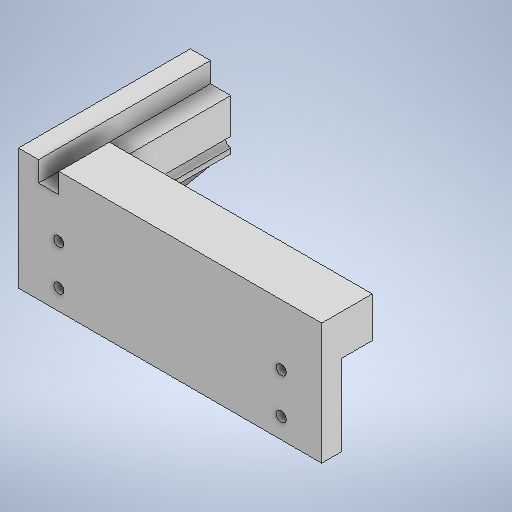
# Autodesk Inventor part: NewModuleConnectorRight
Saved by Autodesk Inventor 2025.3 (Build 293356000, 356)
## iProperties
Created: 2025-05-03
Part Number: NewModuleConnectorRight
Material: 일반
Document SubType Name: Modeling
Designer: SEON
Density: 1 g/cm^3
Appearance: 기본값
Author: SEON
## iProperties of the stored document NewModuleConnectorLeft_3D 인쇄.ipt
Created: 2025-05-03
Part Number: NewModuleConnectorLeft_3D 인쇄
Material: 일반
Document SubType Name: Modeling
Designer: SEON
Density: 1 g/cm^3
Appearance: 기본값
Author: SEON
Autodesk Inventor part; units mm, degrees
ref_plane "YZ Plane" through (0, 0, 0) normal (1, 0, 0) x (0, 1, 0)
ref_plane "XZ Plane" through (0, 0, 0) normal (0, 1, 0) x (-1, 0, 0)
ref_plane "XY Plane" through (0, 0, 0) normal (0, 0, 1) x (1, 0, 0)
sketch "스케치1" plane through (0, 0, 0) normal (0, 0, 1) x (1, 0, 0)
  line L0 (0, 0) -> (150, 0)
  line L1 (150, 0) -> (150, 60)
  line L2 (150, 60) -> (0, 60)
  line L3 (0, 60) -> (0, 0)
  circle A0 centre (20, 30) radius 2.5
  circle A1 centre (20, 10) radius 2.5
  circle A2 centre (130, 30) radius 2.5
  circle A3 centre (130, 10) radius 2.5
  line L4 (10, 60) -> (10, 0)
  line L5 (20, 60) -> (20, 50)
  line L6 (20, 50) -> (10, 50)
  line L7 (20, 50) -> (20, 25)
  line L8 (20, 25) -> (10, 25)
  line L9 (10, 15) -> (0, 15)
  line L10 (20, 40) -> (150, 40)
  point P0 (20, 27.5)
  point P1 (20, 32.5)
  dimension "d0" = 5
  dimension "d1" = 30
  dimension "d2" = 20
  dimension "d3" = 20
  dimension "d4" = 150
  dimension "d5" = 20
  dimension "d6" = 60
  dimension "d7" = 10
  dimension "d8" = 10
  dimension "d9" = 10
  dimension "d10" = 10
  dimension "d11" = 25
  dimension "d16" = 10
  dimension "d19" = 20
  constraints: 22 end point, 9 point on line, 6 perpendicular, 4 centre point, 3 equal radius, 2 horizontal alignment, 2 parallel, 2 vertical alignment, 1 horizontal, 1 vertical
  measures "d0" diameter of A0
  measures "d1" distance from line of L2 A0.centre
  measures "d2" distance of A0.centre A1.centre
  measures "d3" distance from line of A2.centre L1
  measures "d4" distance between parallel lines of L3 L1
  measures "d5" distance from line of L3 A1.centre
  measures "d6" distance of L2.end L0.start
  measures "d7" distance between parallel lines of L3 L4
  measures "d8" distance of L5.end L6.end
  measures "d9" distance of L5.start L5.end
  measures "d10" distance of L7.end L8.end
  measures "d11" distance of L5.end L7.end
  measures "d16" distance between parallel lines of L8 L9
  measures "d19" distance of L1.end L10.end
extrude "돌출1" add sketch "스케치1" along normal blind 10 contours L3 L9 L4 L0 | L4 L8 L7 A0 L10 L1 L0 | L3 L2 L4 L9 | L10 L7 L5 L2 L1 | L4 L6 L7 A0 L8
extrude "돌출2" add sketch "스케치1" against normal blind 75 contours L3 L2 L4 L9 | L4 L6 L7 A0 L8
sketch "스케치2" plane through (0, 0, 10) normal (-1, 0, 0) x (0, 0, -1)
  line L0 (0, -60) -> (0, 0) projected
  line L1 (10, 0) -> (0, 0) projected
  line L2 (10, -15) -> (10, 0) projected
  line L3 (10, -15) -> (85, -15) projected
  line L4 (85, -15) -> (85, -60) projected
  line L5 (85, -15) -> (10, 0)
  line L6 (85, -60) -> (0, -60) projected
  point P0 (0, -2)
  constraints: 2 end point
extrude "돌출3" add sketch "스케치2" against normal up to surface (10 mm away)
extrude "돌출4" add sketch "스케치1" against normal blind 15 contours L10 L7 L5 L2 L1
